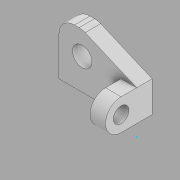
# Autodesk Inventor part: Lab2A01209499P15
Saved by Autodesk Inventor 2020 (Build 240168000, 168)
## iProperties
Created: 2019-08-22
Part Number: Lab2A01209499P15
Material: Genérico
Document SubType Name: Modeling
Designer: gerar
Density: 1 g/cm^3
Appearance: Valor por defecto
Author: gerar
Autodesk Inventor part; units mm, degrees
ref_plane "YZ Plane" through (0, 0, 0) normal (1, 0, 0) x (0, 1, 0)
ref_plane "XZ Plane" through (0, 0, 0) normal (0, 1, 0) x (-1, 0, 0)
ref_plane "XY Plane" through (0, 0, 0) normal (0, 0, 1) x (1, 0, 0)
sketch "Boceto1" plane through (0, 0, 0) normal (0, 0, 1) x (1, 0, 0)
  line L0 (-5, -3.5) -> (5, -3.5)
  line L1 (5, -3.5) -> (5, 0.5)
  line L2 (-2.4105, 3.5) -> (-3, 3.5)
  line L3 (-5, 1.5) -> (-5, -3.5)
  line L4 (-5, -3.5) -> (5, 3.5) construction
  line L5 (5, -3.5) -> (-5, 3.5) construction
  arc A0 (-3, 3.5) -> (-5, 1.5) centre (-3, 1.5) ccw
  line L6 (-1.6227, 3.3383) -> (5, 0.5)
  circle A1 centre (-2, 0.5) radius 1.25
  arc A2 (-1.6227, 3.3383) -> (-2.4105, 3.5) centre (-2.4105, 1.5) ccw
  point P0 (0, 0)
  point P1 (-2, 3.5)
  dimension "d0" = 10
  dimension "d1" = 7
  dimension "d2" = 2
  dimension "d3" = 7
  dimension "d4" = 3
  dimension "d5" = 2.5
  dimension "d6" = 3
  dimension "d7" = 4
  dimension "d10" = 2
  constraints: 14 end point, 6 point on line, 4 point on circle, 4 tangent, 3 centre point, 2 midpoint, 2 parallel, 1 horizontal, 1 perpendicular
  measures "d0" distance of L5.end L4.end
  measures "d1" distance of L4.end L0.end
  measures "d2" radius of A0
  measures "d3" distance of point (-2, 3.5) L4.end
  measures "d4" distance of L1.end L4.end
  measures "d5" diameter of A1
  measures "d6" distance from line of L3 A1.centre
  measures "d7" distance from line of L0 A1.centre
  measures "d10" radius of A2
extrude "Extrusión1" add sketch "Boceto1" along normal blind 2
sketch "Boceto2" plane through (5, -3.5, 0) normal (1, 0, 0) x (0, 0, -1)
  line L0 (0, 0) -> (-2, 0) projected
  line L1 (0, 0) -> (-4, 0)
  line L2 (-6, 2) -> (-6, 2)
  line L3 (-4, 4) -> (0, 4)
  line L4 (0, 4) -> (0, 0)
  circle A0 centre (-4, 2) radius 1
  arc A1 (-4, 4) -> (-6, 2) centre (-4, 2) ccw
  arc A2 (-6, 2) -> (-4, 0) centre (-4, 2) ccw
  point P0 (0, 3.5)
  point P1 (-6, 4)
  point P2 (-6, 0)
  dimension "d11" = 6
  dimension "d12" = 4
  dimension "d13" = 2
  dimension "d14" = 2
  dimension "d15" = 2
  dimension "d16" = 2
  constraints: 8 end point, 4 point on circle, 4 point on line, 4 tangent, 3 centre point, 2 parallel, 1 concentric, 1 horizontal, 1 perpendicular
  measures "d11" distance of point (-6, 4) L3.end
  measures "d12" distance of point (-6, 0) point (-6, 4)
  measures "d13" diameter of A0
  measures "d14" distance from line of L1 A0.centre
  measures "d15" distance from line of L2 A0.centre
  measures "d16" radius of A1
extrude "Extrusión2" add sketch "Boceto2" against normal blind 2
sketch "Boceto3" plane through (3, -3.5, 0) normal (-1, 0, 0) x (0, 0, -1)
  point P0 (0, 3.5)
